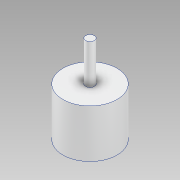
# Autodesk Inventor part: Rotar
Saved by Autodesk Inventor 2020 (Build 240168000, 168)
## iProperties
Created: 2019-08-30
Part Number: Rotar
Material: アルミニウム 6061
Document SubType Name: Modeling
Designer: Ryohei
Density: 2.7 g/cm^3
Appearance: アルミニウム - フラット
Mass: 242.557 g
Surface Area: 120.519 cm^2
Volume: 89.8361 cm^3
Author: Ryohei
Autodesk Inventor part; units mm, degrees
ref_plane "YZ Plane" through (0, 0, 0) normal (1, 0, 0) x (0, 1, 0)
ref_plane "XZ Plane" through (0, 0, 0) normal (0, 1, 0) x (-1, 0, 0)
ref_plane "XY Plane" through (0, 0, 0) normal (0, 0, 1) x (1, 0, 0)
sketch "スケッチ7" plane through (0, 0, 0) normal (0, 1, 0) x (-1, 0, 0)
  circle A0 centre (0, 0) radius 25
  dimension "d28" = 50
  constraints: 1 centre point, 1 coincident
  measures "d28" diameter of A0
extrude "押し出し4" add sketch "スケッチ7" along normal blind 44.5
sketch "スケッチ8" plane through (0, 44.5, 0) normal (0, 1, 0) x (1, 0, 0)
  circle A0 centre (0, 0) radius 4
  dimension "d31" = 8
  constraints: 1 centre point, 1 coincident
  measures "d31" diameter of A0
extrude "押し出し5" add sketch "スケッチ8" along normal blind 36.7
sketch "スケッチ9" plane through (0, 0, 0) normal (0, -1, 0) x (1, 0, 0)
  line L0 (0, 0) -> (7.0711, -7.0711)
  line L1 (0, 0) -> (10, 0) construction
  point P0 (7.0711, 7.0711)
  point P1 (-7.0711, 7.0711)
  point P2 (-7.0711, -7.0711)
  dimension "d34" = 10
  dimension "d35" = 45
  dimension "d38" = 360
  constraints: 4 end point, 1 coincident, 1 equal length, 1 horizontal, 5 other
  measures "d34" distance of L0.start L0.end
  measures "d35" angle of L0 L1
hole "穴2" at (7.0711, 0, -7.0711) at (7.0711, 0, 7.0711) at (-7.0711, 0, 7.0711) at (-7.0711, 0, -7.0711) direction (0, 1, 0) diameter 2.459 depth 8.8 tip angle 118 thread size "M3x0.5" class "6H" standard "ISO Metric profile"
sketch "スケッチ11" plane through (0, 0, 0) normal (0, -1, 0) x (1, 0, 0)
  circle A0 centre (0, 0) radius 7
  dimension "d52" = 14
  constraints: 1 centre point, 1 coincident
  measures "d52" diameter of A0
extrude "押し出し7" add sketch "スケッチ11" along normal blind 2
